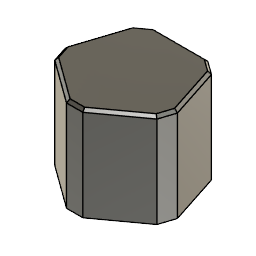
bird thing_v1 (Autodesk Fusion 360 design; units mm, degrees)
Autodesk Fusion 360 part; units mm, degrees
sketch "Sketch1" plane through (0, 0, 0) normal (0, 0, 1) x (1, 0, 0)
  line L0 (-29.563, 30.3671) -> (-41.7663, -7.1908)
  line L1 (-38.0163, -18.7321) -> (-6.0676, -41.9442)
  line L2 (6.0676, -41.9442) -> (38.0163, -18.7321)
  line L3 (41.7663, -7.1908) -> (29.563, 30.3671)
  line L4 (19.7453, 37.5) -> (-19.7453, 37.5)
  line L5 (-29.563, 30.3671) -> (-19.7453, 37.5)
  line L6 (-41.7663, -7.1908) -> (-38.0163, -18.7321)
  line L7 (-6.0676, -41.9442) -> (6.0676, -41.9442)
  line L8 (38.0163, -18.7321) -> (41.7663, -7.1908)
  line L9 (29.563, 30.3671) -> (19.7453, 37.5)
  point P0 (-27.2453, 37.5)
  point P1 (-44.0839, -14.3237)
  point P2 (0, -46.3525)
  point P3 (44.0839, -14.3237)
  point P4 (27.2453, 37.5)
  constraint coincident P0 L0
  constraint coincident P0 L4
  constraint coincident P1 L0
  constraint coincident P1 L1
  constraint coincident P2 L1
  constraint coincident P2 L2
  constraint coincident P3 L2
  constraint coincident P3 L3
  constraint coincident P4 L3
  constraint coincident P4 L4
extrude "Extrude1" add sketch "Sketch1" along normal blind 70
sketch "Sketch2" plane through (0, 0, 0) normal (0, 0, -1) x (1, 0, 0)
  line L0 (-41.7663, 7.1908) -> (-29.563, -30.3671)
  line L1 (-29.563, -30.3671) -> (-19.7453, -37.5)
  line L2 (-19.7453, -37.5) -> (19.7453, -37.5)
  line L3 (19.7453, -37.5) -> (29.563, -30.3671)
  line L4 (29.563, -30.3671) -> (41.7663, 7.1908)
  line L5 (41.7663, 7.1908) -> (38.0163, 18.7321)
  line L6 (38.0163, 18.7321) -> (6.0676, 41.9442)
  line L7 (6.0676, 41.9442) -> (-6.0676, 41.9442)
  line L8 (-6.0676, 41.9442) -> (-38.0163, 18.7321)
  line L9 (-38.0163, 18.7321) -> (-41.7663, 7.1908)
  circle A0 centre (0, 0) radius 3.5
  dimension "d13" = 7
  constraint coincident A0.centre origin
  measures "d13" diameter of A0
extrude "Extrude2" cut sketch "Sketch2" against normal blind 11 contours A0
chamfer "Chamfer1" distance 2 angle 45 1 faces at (-0.7952, -10.1031, 70)
